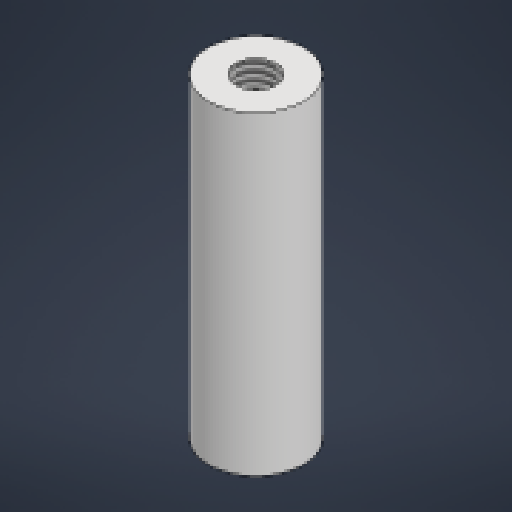
# Autodesk Inventor part: STOCK,REVERSER,STANDOFF
Saved by Autodesk Inventor 2026.1 (Build 301233020, 233B)
## iProperties
Created: 2026-04-01
Part Number: STOCK,REVERSER,STANDOFF
Material: Generic
Document SubType Name: Modeling
Designer: Owen L
Mass: 2.01749 g
Surface Area: 13.3376 cm^2
Volume: 2.01749 cm^3
Density: 1 g/cm^3
Appearance: Default
Author: Owen L
Autodesk Inventor part; units mm, degrees
ref_plane "YZ Plane" through (0, 0, 0) normal (1, 0, 0) x (0, 1, 0)
ref_plane "XZ Plane" through (0, 0, 0) normal (0, 1, 0) x (-1, 0, 0)
ref_plane "XY Plane" through (0, 0, 0) normal (0, 0, 1) x (1, 0, 0)
sketch "Sketch1" plane through (0, 0, 0) normal (0, 1, 0) x (-1, 0, 0)
  circle A0 centre (0, 0) radius 4.7625
  dimension "d0" = 9.525
  constraints: 1 centre point, 1 coincident
  measures "d0" diameter of A0
extrude "Extrusion1" add sketch "Sketch1" along normal mid plane 31.7475
sketch "Sketch2" plane through (0, -15.8737, 0) normal (0, -1, 0) x (1, 0, 0)
  point P0 (0, 0)
  point P1 (0, 0)
  constraints: 1 coincident
hole "Hole1" at (0, -15.8737, 0) direction (0, 1, 0) diameter 3.9624 depth 9.525 tip angle 118 thread size "10-32 UNF" class "2B" standard "ANSI Unified Screw Threads"
mirror "Mirror1" about plane through (0, 0, 0) normal (0, 1, 0) of "Hole1"
body "Solid1"
